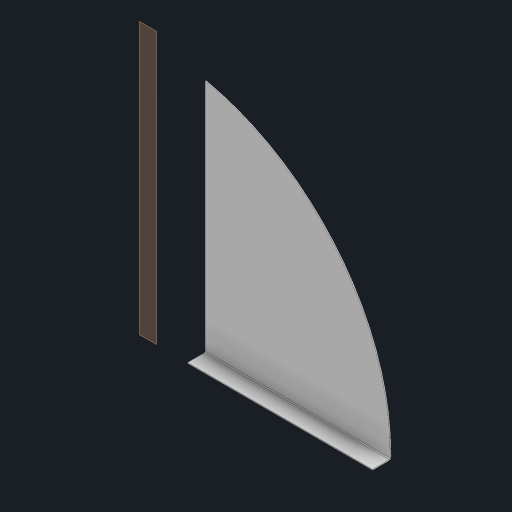
# Autodesk Inventor part: CHAPA_7
Saved by Autodesk Inventor 2024.3 (Build 283343000, 343)
## iProperties
Created: 2024-07-02
Part Number: CHAPA_7
Material: Generic
Document SubType Name: Sheet Metal
Designer: Niler
Density: 1 g/cm^3
Sheet Metal Rule: Default_mm
Appearance: Default
Author: Niler
Autodesk Inventor part; units mm, degrees
ref_plane "YZ Plane" through (0, 0, 0) normal (1, 0, 0) x (0, 1, 0)
ref_plane "XZ Plane" through (0, 0, 0) normal (0, 1, 0) x (-1, 0, 0)
ref_plane "XY Plane" through (0, 0, 0) normal (0, 0, 1) x (1, 0, 0)
ref_plane "Work Plane1" through (0, 0, 0) normal (0, 0, 1) x (1, 0, 0)
sketch "Sketch1" plane through (0, 0, 0) normal (0, 0, 1) x (1, 0, 0)
  arc A0 (381.5, 18.5) -> (0, 400) centre (0, 18.5) ccw
  line L0 (381.5, 18.5) -> (81.5, 18.5)
  line L1 (81.5, 18.5) -> (81.5, 391.1929)
  line L2 (81.5, 18.5) -> (381.5, 18.5)
  line L3 (381.5, 18.5) -> (381.5, -1.5)
  line L4 (381.5, -1.5) -> (81.5, -1.5)
  line L5 (81.5, -1.5) -> (81.5, 18.5)
  point P0 (0, 0)
  dimension "d0" = 300
  dimension "d2" = 20
  measures "d0" distance of L0.start L0.end
  measures "d2" distance of L4.end L0.end
extrude "Plate1" add sketch "Sketch1" along normal blind 1.5
sketch "Sketch2" plane through (0, 0, 1.5) normal (0, 0, 1) x (1, 0, 0)
  arc A0 (381.5, 18.5) -> (81.5, 391.1929) centre (0, 18.5) ccw projected
  line L0 (81.5, -1.5) -> (81.5, 391.1929) projected
  line L1 (381.5, -1.5) -> (81.5, -1.5) projected
  line L2 (381.5, 18.5) -> (381.5, -1.5) projected
  line L3 (81.5, 8.5) -> (381.5, 8.5)
  point P0 (0, 0)
  dimension "d3" = 10
  constraints: 2 end point, 1 midpoint, 1 perpendicular, 1 point on line
  measures "d3" distance between parallel lines of L1 L3
extrude "Extrusion1" cut sketch "Sketch2" against normal through all contours L2 L1 L0 L3
sketch "Sketch3" plane through (381.5, 10, 0) normal (0, -1, 0) x (1, 0, 0)
  line L0 (-300, 0) -> (0, 0)
  line L1 (0, 0) -> (0, 30)
  line L2 (0, 30) -> (-300, 30)
  line L3 (-300, 30) -> (-300, 0)
  constraints: 6 end point, 1 horizontal, 1 perpendicular, 1 vertical
edge flange "Flange1" height 30 angle 90 thickness 1.5 bend radius 1.5 thickness toward (0, -1, 0) relief tear relief width 1.5 relief depth 0.75 edges at (231.5, 8.5, 1.5) wall of the first edge with corners at (81.5, 10, 0) (381.5, 10, 0) (381.5, 10, 30) (81.5, 10, 30)
bend "Bend1"
corner "Corner1"
equation "\"d1\" = Thickness"
equation "\"d6\" = BendReliefWidth"
equation "\"d7\" = BendReliefDepth"
equation "\"d8\" = MinimumRemnant"
equation "\"d9\" = TransitionRadius"
equation "\"d12\" = BendRadius"
equation "\"d13\" = CornerReliefSize"
equation "\"d14\" = GapSize"
equation "\"d15\" = JacobiRadiusSize"
equation "\"BendRadius\" = Thickness"
equation "\"BendReliefWidth\" = Thickness"
equation "\"BendReliefDepth\" = 0.5 * Thickness"
equation "\"CornerReliefSize\" = 4 * Thickness"
equation "\"MinimumRemnant\" = 2 * Thickness"
equation "\"TransitionRadius\" = BendRadius"
equation "\"JacobiRadiusSize\" = BendRadius"
equation "\"GapSize\" = Thickness"
equation "\"Thickness\" = 1.5"
body "Solid1"
